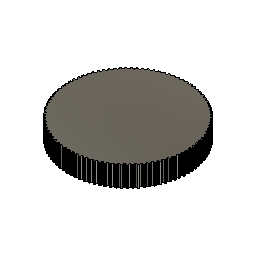
gear_93z (Autodesk Fusion 360 design; units mm, degrees)
Autodesk Fusion 360 part; units mm, degrees
sketch "Sketch1" plane through (0, 0, 0) normal (0, 0, 1) x (1, 0, 0) in component "gt2 pulley"
  circle A0 centre (0, 0) radius 29.6028 construction
  circle A1 centre (0, 0) radius 28.5988 construction
  line L0 (0, 0) -> (0, 29.6028) construction
  line L1 (0, 0) -> (0.9998, 29.5859) construction
  line L2 (0, 0) -> (1.4043, 29.5695) construction
  circle A2 centre (0, 0) radius 29.3488 construction
  arc A3 (0.3975, 29.2132) -> (0.4763, 28.9144) centre (1.3922, 29.3158) ccw
  circle A4 centre (0, 0) radius 29.1988 construction
  arc A5 (0.2495, 29.3478) -> (0, 29.3488) centre (0, 0) ccw
  arc A6 (0.3975, 29.2132) -> (0.2495, 29.3478) centre (0.2483, 29.1978) ccw
  arc A7 (0.4763, 28.9144) -> (0.9659, 28.5825) centre (0.9846, 29.1372) ccw
  arc A8 (0, 29.3488) -> (-0.2495, 29.3478) centre (0, 0) ccw
  arc A9 (-0.2495, 29.3478) -> (-0.3975, 29.2132) centre (-0.2483, 29.1978) ccw
  arc A10 (-0.4763, 28.9144) -> (-0.3975, 29.2132) centre (-1.3922, 29.3158) ccw
  arc A11 (-0.9658, 28.5825) -> (-0.4763, 28.9144) centre (-0.9846, 29.1372) ccw
  arc A12 (0.9659, 28.5825) -> (-0.9659, 28.5825) centre (0, 0) ccw
  point P0 (1.3922, 29.3158)
  point P1 (0, 29.3488)
  dimension "d18" = 59.2056
  dimension "d19" = 1.935
  dimension "d22" = 1.004
  dimension "d24" = 0.75
  dimension "d26" = 1
  dimension "d27" = 0.15
  dimension "d28" = 0.15
  dimension "d47" = 0.555
  dimension "d52" = 3.812
  constraint coincident A0.centre A1.centre
  constraint coincident A0 L0.end
  constraint vertical L0
  constraint coincident A0 L1.end
  constraint coincident A0 L2.end
  constraint concentric A1 A2
  constraint coincident A1 A7.end
  constraint coincident L1 A7.end
  constraint coincident A2 P0
  constraint coincident L2 P0
  constraint coincident P0 A3.centre
  constraint coincident A2 P1
  constraint coincident L0 P1
  constraint concentric A2 A4
  constraint coincident P1 A5.end
  constraint coincident A4 A6.centre
  constraint coincident A3.start A6.start
  constraint tangent A3 A6
  constraint tangent A3 A7
  constraint symmetric L0 A7.end A12.end
  constraint symmetric L0 A3.start A9.end
  constraint symmetric L0 A3.end A10.start
  constraint symmetric L0 A3 A10
  constraint symmetric L0 A5.start A8.end
  constraint symmetric L0 P1 A5.end
  constraint symmetric L0 A5 A8
  constraint symmetric L0 A6 A9
  constraint symmetric L0 A7 A11
  constraint coincident A1 A11.start
  constraint tangent A1 A7
  constraint coincident L1 A7.centre
  measures "d18" diameter of A0
  measures "d19" angle of L0 L1
  measures "d22" distance of A0 A1
  measures "d24" distance of A1 A2
  measures "d26" radius of A3
  measures "d27" distance of A2 A4
  measures "d28" radius of A6
  measures "d47" radius of A7
extrude "Extrude1" add sketch "Sketch1" along normal blind 10 makes body 1
pattern_circular "C-Pattern1" count 93 over 360 about axis through (0, 0, 1.75) along (0, 0, 1) of bodies 1 makes body 2 at (-2.0377, 28.5261, 6.6667) makes body 3 at (-4.3836, 28.2609, 6.6667) makes body 4 at (-5.019, 28.155, 6.6667) makes body 5 at (-7.7383, 27.532, 6.6667) makes body 6 at (-9.5793, 26.9468, 6.6667) makes body 7 at (-10.5838, 26.5683, 3.3333) makes body 8 at (-13.122, 25.4107, 6.6667) makes body 9 at (-14.8076, 24.4669, 6.6667) makes body 10 at (-15.7153, 23.894, 3.3333) makes body 11 at (-18.465, 21.8389, 6.6667) makes body 12 at (-19.8972, 20.5425, 6.6667) makes body 13 at (-20.2034, 20.2414, 3.3333) makes body 14 at (-21.5238, 18.8313, 3.3333) makes body 15 at (-22.746, 17.3353, 3.3333) makes body 16 at (-24.3268, 15.0366, 6.6667) makes body 17 at (-25.5808, 12.7872, 6.6667) makes body 18 at (-25.77, 12.4017, 3.3333) makes body 19 at (-26.5484, 10.6336, 6.6667) makes body 20 at (-27.2057, 8.8171, 6.6667) makes body 21 at (-27.7389, 6.9603, 3.3333) makes body 22 at (-28.1455, 5.0718, 3.3333) makes body 23 at (-28.5504, 1.663, 6.6667) makes body 24 at (-28.5964, 0.3758, 6.6667) makes body 25 at (-28.5903, -0.6976, 3.3333) makes body 26 at (-28.478, -2.6262, 3.3333) makes body 27 at (-28.0866, -5.3883, 6.6667) makes body 28 at (-27.8646, -6.4386, 3.3333) makes body 29 at (-26.8924, -9.7308, 6.6667) makes body 30 at (-26.7433, -10.1335, 3.3333) makes body 31 at (-25.9982, -11.9159, 3.3333) makes body 32 at (-25.1344, -13.6438, 3.3333) makes body 33 at (-23.8051, -15.8495, 6.6667) makes body 34 at (-22.1476, -18.0935, 6.6667) makes body 35 at (-21.453, -18.9119, 6.6667) makes body 36 at (-20.5797, -19.8587, 3.3333) makes body 37 at (-19.1921, -21.2027, 3.3333) makes body 38 at (-17.035, -22.9717, 6.6667) makes body 39 at (-14.8994, -24.4111, 6.6667) makes body 40 at (-13.2175, -25.3612, 6.6667) makes body 41 at (-11.4752, -26.1957, 6.6667) makes body 42 at (-11.0805, -26.365, 3.3333) makes body 43 at (-8.459, -27.3192, 6.6667) makes body 44 at (-5.9671, -27.9694, 6.6667) makes body 45 at (-5.5465, -28.0558, 3.3333) makes body 46 at (-3.6398, -28.3663, 3.3333) makes body 47 at (-1.7165, -28.5473, 3.3333) makes body 48 at (0.2147, -28.598, 3.3333) makes body 49 at (3.6397, -28.3663, 6.6667) makes body 50 at (4.0652, -28.3084, 3.3333) makes body 51 at (7.2202, -27.6724, 6.6667) makes body 52 at (9.2752, -27.053, 6.6667) makes body 53 at (9.6804, -26.9106, 3.3333) makes body 54 at (12.835, -25.5569, 6.6667) makes body 55 at (13.2174, -25.3613, 6.6667) makes body 56 at (14.8993, -24.4111, 3.3333) makes body 57 at (17.2069, -22.8433, 6.6667) makes body 58 at (18.052, -22.1815, 3.3333) makes body 59 at (19.5083, -20.9122, 6.6667) makes body 60 at (21.3104, -19.0725, 6.6667) makes body 61 at (23.0673, -16.9054, 6.6667) makes body 62 at (23.3185, -16.5571, 3.3333) makes body 63 at (24.3831, -14.9451, 3.3333) makes body 64 at (25.9981, -11.916, 6.6667) makes body 65 at (26.1741, -11.5242, 3.3333) makes body 66 at (26.8924, -9.7309, 3.3333) makes body 67 at (27.6587, -7.2723, 6.6667) makes body 68 at (28.0866, -5.3885, 6.6667) makes body 69 at (28.3007, -4.1183, 3.3333) makes body 70 at (28.5673, -1.3414, 6.6667) makes body 71 at (28.5976, -0.2684, 3.3333) makes body 72 at (28.5504, 1.6629, 3.3333) makes body 73 at (28.2851, 4.2245, 6.6667) makes body 74 at (27.8886, 6.3339, 6.6667) makes body 75 at (27.2058, 8.817, 6.6667) makes body 76 at (26.7812, 10.0331, 6.6667) makes body 77 at (26.1307, 11.6223, 6.6667) makes body 78 at (25.2865, 13.3599, 6.6667) makes body 79 at (24.6593, 14.4849, 3.3333) makes body 80 at (22.7461, 17.3352, 6.6667) makes body 81 at (21.5239, 18.8312, 6.6667) makes body 82 at (21.2387, 19.1523, 3.3333) makes body 83 at (19.2716, 21.1305, 6.6667) makes body 84 at (17.2926, 22.7785, 6.6667) makes body 85 at (16.9486, 23.0356, 3.3333) makes body 86 at (14.6236, 24.5773, 6.6667) makes body 87 at (13.1221, 25.4107, 6.6667) makes body 88 at (11.1794, 26.3232, 6.6667) makes body 89 at (8.7661, 27.2222, 6.6667) makes body 90 at (7.5315, 27.5893, 6.6667) makes body 91 at (6.4909, 27.8525, 3.3333) makes body 92 at (4.5957, 28.2271, 3.3333) makes body 93 at (2.6796, 28.473, 3.3333)
sketch "Sketch2" plane through (0, 0, 10) normal (0, 0, 1) x (-1, 0, 0)
  arc A0 (-6.2699, -28.5351) -> (-6.1521, -28.6968) centre (-6.1207, -28.5501) ccw
  arc A1 (-6.1521, -28.6968) -> (-5.6632, -28.7972) centre (0, 0) ccw
  arc A2 (-5.6632, -28.7972) -> (-5.4912, -28.6952) centre (-5.6342, -28.6501) ccw
  arc A3 (-5.3539, -28.4184) -> (-5.4912, -28.6952) centre (-4.5375, -28.9959) ccw
  arc A4 (-4.8076, -28.1918) -> (-5.3539, -28.4184) centre (-4.9008, -28.739) ccw
  arc A5 (-6.6997, -27.803) -> (-4.8076, -28.1918) centre (0, 0) ccw
  arc A6 (-6.287, -28.2267) -> (-6.6997, -27.803) centre (-6.8298, -28.3425) ccw
  arc A7 (-6.2699, -28.5351) -> (-6.287, -28.2267) centre (-7.265, -28.4354) ccw
  circle A8 centre (0, 0) radius 28.5988
  constraint concentric A1 A8
extrude "Extrude2" add sketch "Sketch2" against normal blind 10 contours A5 A8 bodies 1 2 3 4 5 6 7 8 9 10 11 12 13 14 15 16 17 18 19 20 21 22 23 24 25 26 27 28 29 30 31 32 33 34 35 36 37 38 39 40 41 42 43 44 45 46 47 48 49 50 51 52 53 54 55 56 57 58 59 60 61 62 63 64 65 66 67 68 69 70 71 72 73 74 75 76 77 78 79 80 81 82 83 84 85 86 87 88 89 90 91 92 93
extrude "Extrude4" [suppressed] in component "gt2 pulley"
pattern_circular "C-Pattern7" [suppressed] in component "gt2 pulley"
extrude "Extrude3" [suppressed] in component "gt2 pulley"
pattern_circular "C-Pattern6" [suppressed] in component "gt2 pulley"
extrude "Extrude2'" [suppressed] in component "gt2 pulley"
pattern_circular "C-Pattern5" [suppressed] in component "gt2 pulley"
extrude "Extrude1'" [suppressed] in component "gt2 pulley"
pattern_circular "C-Pattern4" [suppressed] in component "gt2 pulley"
pattern_circular "C-Pattern3" [suppressed] in component "gt2 pulley"
pattern_circular "C-Pattern2" [suppressed] in component "gt2 pulley"
pattern_circular "C-Pattern1'" [suppressed] in component "gt2 pulley"
copy_body "Body->Comp1" [suppressed] in component "Component"
copy_body "Body->Comp2" [suppressed] in component "Component'"
copy_body "Body->Comp3" [suppressed] in component "Component''"
copy_body "Body->Comp4" [suppressed] in component "Component'''"
copy_body "Body->Comp5" [suppressed] in component "Component''''"
copy_body "Body->Comp6" [suppressed] in component "Component'''''"
copy_body "Body->Comp7" [suppressed] in component "Component''''''"
copy_body "Body->Comp8" [suppressed] in component "Component'''''''"
copy_body "Body->Comp9" [suppressed] in component "Component''''''''"
copy_body "Body->Comp10" [suppressed] in component "Component'''''''''"
copy_body "Body->Comp11" [suppressed] in component "Component''''''''''"
copy_body "Body->Comp12" [suppressed] in component "Component'''''''''''"
copy_body "Body->Comp13" [suppressed] in component "Component''''''''''''"
copy_body "Body->Comp14" [suppressed] in component "Component'''''''''''''"
copy_body "Body->Comp15" [suppressed] in component "Component''''''''''''''"
copy_body "Body->Comp16" [suppressed] in component "Component'''''''''''''''"
copy_body "Body->Comp17" [suppressed] in component "Component''''''''''''''''"
copy_body "Body->Comp18" [suppressed] in component "Component'''''''''''''''''"
copy_body "Body->Comp19" [suppressed] in component "Component''''''''''''''''''"
copy_body "Body->Comp20" [suppressed] in component "Component'''''''''''''''''''"
component "gt2 pulley" placed x (1, 0, 0) y (0, 1, 0) z (0, 0, 1) at (0, 0, 0)
equation "NumTeeth = 93" comment "min 20"
equation "ToothPitch = 2 mm"
equation "PullyDia = NumTeeth * ToothPitch / PI"
equation "ToothAng = ( ( 360 / NumTeeth ) * 1 deg )"
equation "TransOffsetAngle = ToothAng * 0.2"
equation "Sholulder_Radius = 0.15 mm"
equation "Root_Radius = 0.555 mm"
equation "TransRadius = 1 mm"
equation "ToolHeight = 0.75 mm"
equation "PLD = 0.254 mm"
equation "d18 = PullyDia"
equation "d19 = ToothAng / 2"
equation "d22 = PLD + ToolHeight"
equation "d24 = ToolHeight"
equation "d26 = TransRadius"
equation "d27 = Sholulder_Radius"
equation "d31 = NumTeeth"
equation "d33 = NumTeeth"
equation "d35 = NumTeeth"
equation "d37 = NumTeeth"
equation "d41 = NumTeeth"
equation "d45 = NumTeeth"
equation "d47 = Root_Radius"
equation "d50 = NumTeeth"
